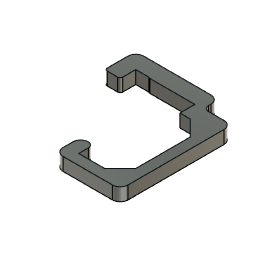
Single motor Holder v5 (Body) (Autodesk Fusion 360 design; units mm, degrees)
Autodesk Fusion 360 part; units mm, degrees
note: some values were not read from the file. Set by a fixed rule: which sketch regions a step uses.
sketch "Sketch1" plane through (0, 0, 0) normal (0, 0, 1) x (1, 0, 0)
  line L0 (60.0013, 14) -> (60.0013, 15)
  arc A0 (60.0013, 14) -> (62.0013, 12) centre (62.0013, 14) ccw
  line L1 (51, -27) -> (51, -22.0146)
  line L2 (61, 6) -> (66, 1)
  line L3 (39.0326, 12) -> (39.0326, 11.75)
  line L4 (61, -27) -> (57, -27)
  line L5 (57.0013, 6) -> (61, 6)
  arc A1 (68.0013, -31) -> (71.0013, -28) centre (68.0013, -28) ccw
  line L6 (46, -24.2507) -> (46, -28)
  line L7 (28, 15) -> (28, 6)
  arc A2 (31, 18) -> (28, 15) centre (31, 15) ccw
  line L8 (34, 6) -> (34, 12)
  arc A3 (71.0013, 9) -> (68.0013, 12) centre (68.0013, 9) ccw
  arc A4 (60.0013, 15) -> (57.0013, 18) centre (57.0013, 15) ccw
  arc A5 (46, -28) -> (49, -31) centre (49, -28) ccw
  line L9 (34, 12) -> (39.0326, 12)
  line L10 (68.0013, 12) -> (62.0013, 12)
  line L11 (71.0013, -28) -> (71.0013, 9)
  line L12 (57, 12) -> (57.0013, 12)
  line L13 (39.0326, 11.75) -> (57, 11.75)
  line L14 (49, -31) -> (68.0013, -31)
  line L15 (57.0013, 18) -> (31, 18)
  line L16 (66, 1) -> (66, -22)
  line L17 (28, 6) -> (34, 6)
  line L18 (57, -27) -> (51, -27)
  arc A6 (51, -22.0146) -> (46, -24.2507) centre (49, -24.2507) ccw
  line L19 (66, -22) -> (61, -27)
  line L20 (57.0013, 11.75) -> (57.0013, 6)
  line L21 (57, 11.75) -> (57.0013, 11.75)
  constraint perpendicular L20 L21
extrude "Extrude1" add sketch "Sketch1" along normal blind 5
fillet "Fillet1" radius 1 2 edges at (28, 6, 2.5) (34, 6, 2.5)
fillet "Fillet2" radius 2 1 edges at (51, -22.0146, 2.5)
fillet "Fillet3" radius 1 1 edges at (39.0326, 11.75, 2.5)
sketch "Sketch2" plane through (0, 0, 5) normal (0, 0, 1) x (-1, 0, 0)
  arc A0 (-39.0326, -12) -> (-39.694, -11.75) centre (-39.694, -12.75) ccw
  line L0 (-39.694, -11.75) -> (-57.0013, -11.75)
  line L1 (-57.0013, -11.75) -> (-57.0013, -6)
  line L2 (-57.0013, -6) -> (-61, -6)
  line L3 (-61, -6) -> (-66, -1)
  line L4 (-66, -1) -> (-66, 22)
  line L5 (-66, 22) -> (-61, 27)
  line L6 (-61, 27) -> (-51, 27)
  line L7 (-51, 27) -> (-51, 23.2507)
  arc A1 (-51, 23.2507) -> (-49, 21.2507) centre (-49, 23.2507) ccw
  arc A2 (-49, 21.2507) -> (-46, 24.2507) centre (-49, 24.2507) ccw
  line L8 (-46, 24.2507) -> (-46, 28)
  arc A3 (-46, 28) -> (-49, 31) centre (-49, 28) ccw
  line L9 (-49, 31) -> (-68.0013, 31)
  arc A4 (-68.0013, 31) -> (-71.0013, 28) centre (-68.0013, 28) ccw
  line L10 (-71.0013, 28) -> (-71.0013, -9)
  arc A5 (-71.0013, -9) -> (-68.0013, -12) centre (-68.0013, -9) ccw
  line L11 (-68.0013, -12) -> (-62.0013, -12)
  arc A6 (-60.0013, -14) -> (-62.0013, -12) centre (-62.0013, -14) ccw
  line L12 (-60.0013, -14) -> (-60.0013, -15)
  arc A7 (-60.0013, -15) -> (-57.0013, -18) centre (-57.0013, -15) ccw
  line L13 (-57.0013, -18) -> (-31, -18)
  arc A8 (-31, -18) -> (-28, -15) centre (-31, -15) ccw
  line L14 (-28, -15) -> (-28, -7)
  arc A9 (-28, -7) -> (-29, -6) centre (-29, -7) ccw
  line L15 (-29, -6) -> (-33, -6)
  arc A10 (-33, -6) -> (-34, -7) centre (-33, -7) ccw
  line L16 (-34, -7) -> (-34, -12)
  line L17 (-34, -12) -> (-39.0326, -12)
  line L18 (-66, -1) -> (-67, 0)
  line L19 (-67, 0) -> (-67, 21)
  line L20 (-67, 21) -> (-66, 22)
  constraint coincident L3.end L4.start
  constraint parallel L3 L18
  constraint parallel L4 L19
  constraint coincident L4.end L5.start
  constraint parallel L5 L20
extrude "Extrude2" cut sketch "Sketch2" against normal blind 6 contours L4 L18 L19 L20
sketch "Sketch3" plane through (0, 0, 5) normal (0, 0, 1) x (-1, 0, 0)
  line L0 (-66, -1) -> (-67, 0)
  line L1 (-67, 0) -> (-67, 21)
  line L2 (-67, 21) -> (-61, 27)
  line L3 (-61, 27) -> (-51, 27)
  line L4 (-51, 27) -> (-51, 23.2507)
  arc A0 (-51, 23.2507) -> (-49, 21.2507) centre (-49, 23.2507) ccw
  arc A1 (-49, 21.2507) -> (-46, 24.2507) centre (-49, 24.2507) ccw
  line L5 (-46, 24.2507) -> (-46, 28)
  arc A2 (-46, 28) -> (-49, 31) centre (-49, 28) ccw
  line L6 (-49, 31) -> (-68.0013, 31)
  arc A3 (-68.0013, 31) -> (-71.0013, 28) centre (-68.0013, 28) ccw
  line L7 (-71.0013, 28) -> (-71.0013, -9)
  arc A4 (-71.0013, -9) -> (-68.0013, -12) centre (-68.0013, -9) ccw
  line L8 (-68.0013, -12) -> (-62.0013, -12)
  arc A5 (-60.0013, -14) -> (-62.0013, -12) centre (-62.0013, -14) ccw
  line L9 (-60.0013, -14) -> (-60.0013, -15)
  arc A6 (-60.0013, -15) -> (-57.0013, -18) centre (-57.0013, -15) ccw
  line L10 (-57.0013, -18) -> (-31, -18)
  arc A7 (-31, -18) -> (-28, -15) centre (-31, -15) ccw
  line L11 (-28, -15) -> (-28, -7)
  arc A8 (-28, -7) -> (-29, -6) centre (-29, -7) ccw
  line L12 (-29, -6) -> (-33, -6)
  arc A9 (-33, -6) -> (-34, -7) centre (-33, -7) ccw
  line L13 (-34, -7) -> (-34, -12)
  line L14 (-34, -12) -> (-39.0326, -12)
  arc A10 (-39.0326, -12) -> (-39.694, -11.75) centre (-39.694, -12.75) ccw
  line L15 (-39.694, -11.75) -> (-57.0013, -11.75)
  line L16 (-57.0013, -11.75) -> (-57.0013, -6)
  line L17 (-57.0013, -6) -> (-61, -6)
  line L18 (-61, -6) -> (-66, -1)
